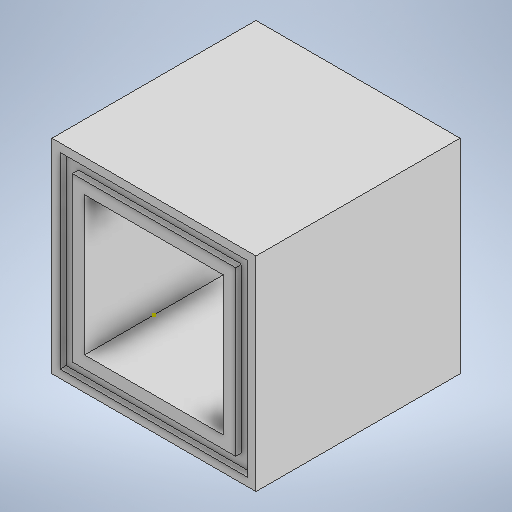
# Autodesk Inventor part: Sweep_0002_001
Saved by Autodesk Inventor 2025.2 (Build 292293000, 293)
## iProperties
Created: 2025-03-26
Part Number: Sweep_0002_001
Material: Genérico
Document SubType Name: Modeling
Designer: lucas
Density: 1 g/cm^3
Appearance: Padrão
Author: lucas
Autodesk Inventor part; units mm, degrees
ref_plane "YZ Plane" through (0, 0, 0) normal (1, 0, 0) x (0, 1, 0)
ref_plane "XZ Plane" through (0, 0, 0) normal (0, 1, 0) x (-1, 0, 0)
ref_plane "XY Plane" through (0, 0, 0) normal (0, 0, 1) x (1, 0, 0)
sketch "Esboço1" plane through (0, 0, 0) normal (0, 0, 1) x (1, 0, 0)
  line L0 (-25, -25) -> (25, -25)
  line L1 (25, -25) -> (25, 25)
  line L2 (25, 25) -> (-25, 25)
  line L3 (-25, 25) -> (-25, -25)
  line L4 (-25, -25) -> (25, 25) construction
  line L5 (25, -25) -> (-25, 25) construction
  line L6 (-17, -17) -> (17, -17)
  line L7 (17, -17) -> (17, 17)
  line L8 (17, 17) -> (-17, 17)
  line L9 (-17, 17) -> (-17, -17)
  line L10 (-17, -17) -> (17, 17) construction
  line L11 (17, -17) -> (-17, 17) construction
  point P0 (0, 0)
  dimension "d0" = 50
  dimension "d2" = 8
  constraints: 24 end point, 4 midpoint, 4 parallel, 4 perpendicular, 2 horizontal
  measures "d0" distance of L2.end L1.end
  measures "d2" distance between parallel lines of L8 L2
extrude "Extrusão1" add sketch "Esboço1" along normal mid plane 50
sketch "Esboço2" plane through (0, 0, 25) normal (0, 0, 1) x (1, 0, 0)
  line L0 (-21.5, -21.5) -> (21.5, -21.5)
  line L1 (21.5, -21.5) -> (21.5, 21.5)
  line L2 (21.5, 21.5) -> (-21.5, 21.5)
  line L3 (-21.5, 21.5) -> (-21.5, -21.5)
  line L4 (-21.5, -21.5) -> (21.5, 21.5) construction
  line L5 (21.5, -21.5) -> (-21.5, 21.5) construction
  line L6 (25, 25) -> (-25, 25) projected
  point P0 (0, 0)
  point P1 (0, 21.5)
  point P2 (0, -21.5)
  point P3 (-21.5, 0)
  point P4 (21.5, 0)
  dimension "d5" = 3.5
  constraints: 12 end point, 6 midpoint, 2 horizontal alignment, 2 parallel, 2 perpendicular, 2 vertical alignment, 1 horizontal
  measures "d5" distance between parallel lines of L6 L2
sketch "Esboço3" plane through (0, 0, 25) normal (0, 0, 1) x (1, 0, 0)
  point P0 (0, 0)
sketch "Esboço8" plane through (0, 0, 0) normal (0, 1, 0) x (-1, 0, 0)
  point P0 (0, 0)
sketch "Esboço9" plane through (0, 0, 0) normal (0, 1, 0) x (-1, 0, 0)
  line L0 (-23, 23.5) -> (-20, 23.5)
  line L1 (-20, 23.5) -> (-20, 26.5)
  line L2 (-20, 26.5) -> (-23, 26.5)
  line L3 (-23, 26.5) -> (-23, 23.5)
  line L4 (25, 25) -> (-25, 25) projected
  line L5 (-23, 23.5) -> (-20, 26.5) construction
  line L6 (-20, 23.5) -> (-23, 26.5) construction
  point P0 (0, 0)
  point P1 (-21.5, 25)
  dimension "d6" = 3
  dimension "d7" = 21.5
  constraints: 12 end point, 2 midpoint, 2 parallel, 2 perpendicular, 1 horizontal, 1 point on line
  measures "d6" distance of L1.end L2.end
  measures "d7" horizontal distance of point (0, 0) point (-21.5, 25)
sweep "Varredura1" cut profiles "Esboço9" path "Esboço2" path curves L1 L0 L3 L2
equation "\"d3\" = d0"
